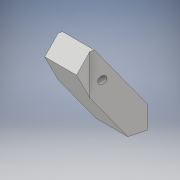
# Autodesk Inventor part: Screen Adapter
Saved by Autodesk Inventor 2017 (Build 210142000, 142)
## iProperties
Created: 2017-04-05
Part Number: Screen Adapter
Material: Generic
Document SubType Name: Modeling
Designer: gilef
Density: 1 g/cm^3
Appearance: Default
Author: gilef
Autodesk Inventor part; units mm, degrees
sketch "Sketch1" plane through (0, 0, 0) normal (0, 0, 1) x (1, 0, 0)
  line L0 (0, 0) -> (5.6109, 21.4027)
  line L1 (5.6109, 21.4027) -> (20.6109, 21.4027)
  line L2 (20.6109, 21.4027) -> (15, 0)
  line L3 (15, 0) -> (21.9438, -13.6515)
  line L4 (21.9438, -13.6515) -> (6.9438, -13.6515)
  line L5 (0, 0) -> (6.9438, -13.6515)
  line L6 (0, 0) -> (0, 15.6682) construction
  dimension "d0" = 138.35
  dimension "d1" = 138.35
  dimension "d2" = 15.316
  dimension "d3" = 22.126
  dimension "d4" = 15
  dimension "d5" = 14.69
  constraints: 14 end point, 2 parallel, 1 horizontal, 1 horizontal alignment, 1 vertical
  measures "d0" angle of L5 L0
  measures "d1" angle of L3 L2
  measures "d2" distance of L0.start L4.end
  measures "d3" distance of L0.start L0.end
  measures "d4" distance of L2.end L0.start
  measures "d5" angle of L6 L0
extrude "Extrusion1" add sketch "Sketch1" along normal blind 40
ref_plane "Work Plane1" through (18.4719, 13.2435, 1) normal (1, 0, 0) x (0, 0, -1)
sketch "Sketch3" plane through (18.4719, 13.2435, 1) normal (1, 0, 0) x (0, 0, -1)
  circle A0 centre (-25.6667, -8.5907) radius 1.75
  line L0 (1, 8.1593) -> (1, -13.2435) projected
  line L1 (-39, -13.2435) -> (-39, 8.1593) projected
  line L2 (1, 8.1593) -> (-39, 8.1593) projected
  dimension "d11" = 3.5
  dimension "d12" = 26.6667
  dimension "d13" = 13.3333
  dimension "d14" = 15
  constraints: 1 centre point
  measures "d11" diameter of A0
  measures "d12" distance from line of L0 A0.centre
  measures "d13" distance from line of L1 A0.centre
  measures "d14" distance edge to line of A0 L2
extrude "Extrusion3" cut sketch "Sketch3" against normal through all
ref_plane "Work Plane9" through (5.6109, 21.4027, 0) normal (0, -0.829, -0.5592) x (1, 0, 0)
ref_plane "Work Plane8" through (21.9438, -13.6515, 40) normal (0, -1, 0) x (1, 0, 0)
ref_plane "Work Plane10" through (5.6109, 16.4285, -3.3552) normal (0, -0.829, -0.5592) x (1, 0, 0)
ref_plane "Work Plane11" through (5.6109, 26.377, 3.3552) normal (0, -0.829, -0.5592) x (1, 0, 0)
split "Split7" plane through (5.6109, 26.377, 3.3552) removes the side toward (0, 0.829, 0.5592)
split "Split8" plane through (5.6109, 16.4285, -3.3552) removes the side toward (0, -0.829, -0.5592)
equation "\"d1\" = d0"
equation "\"d12\" = 2 * d13"
body "Solid1"
